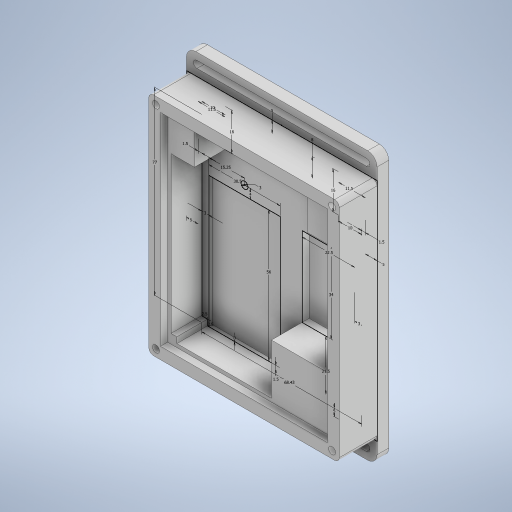
# Autodesk Inventor part: Component_shield_layered
Saved by Autodesk Inventor 2024 (Build 280153000, 153)
## iProperties
Created: 2024-10-22
Part Number: Component_shield_layered
Material: Generic
Document SubType Name: Modeling
Designer: Bruger
Density: 1 g/cm^3
Appearance: Default
Author: Bruger
Autodesk Inventor part; units mm, degrees
ref_plane "YZ Plane" through (0, 0, 0) normal (1, 0, 0) x (0, 1, 0)
ref_plane "XZ Plane" through (0, 0, 0) normal (0, 1, 0) x (-1, 0, 0)
sketch "Sketch1" plane through (0, 0, 0) normal (0, 0, 1) x (1, 0, 0)
  line L0 (0, 0) -> (68.43, 0)
  line L1 (68.43, 0) -> (68.43, 77)
  line L2 (68.43, 77) -> (0, 77)
  line L3 (0, 77) -> (0, 0)
  line L4 (3, 56) -> (33.5, 56)
  line L5 (33.5, 56) -> (33.5, 0)
  line L6 (33.5, 0) -> (3, 0)
  line L7 (3, 0) -> (3, 56)
  line L8 (42.93, 55.5) -> (65.43, 55.5)
  line L9 (65.43, 55.5) -> (65.43, 21.5)
  line L10 (65.43, 21.5) -> (42.93, 21.5)
  line L11 (42.93, 21.5) -> (42.93, 55.5)
  line L12 (-6.5, 90) -> (74.93, 90)
  line L13 (74.93, 90) -> (74.93, -6.5)
  line L14 (74.93, -6.5) -> (-6.5, -6.5)
  line L15 (-6.5, -6.5) -> (-6.5, 90)
  line L16 (-1.5, 85) -> (69.93, 85)
  line L17 (69.93, 85) -> (69.93, -1.5)
  line L18 (69.93, -1.5) -> (-1.5, -1.5)
  line L19 (-1.5, -1.5) -> (-1.5, 85)
  line L20 (42.93, 21.5) -> (68.43, 21.5)
  line L21 (68.43, 21.5) -> (68.43, 0)
  line L22 (68.43, 0) -> (42.93, 0)
  line L23 (42.93, 0) -> (42.93, 21.5)
  line L24 (0, 77) -> (10, 77)
  line L25 (68.43, 77) -> (53.43, 77)
  line L26 (68.43, 67) -> (68.43, 77)
  line L27 (0, 0) -> (2.5, 0)
  line L28 (2.5, 0) -> (2.5, 2.5)
  line L29 (2.5, 2.5) -> (0, 2.5)
  line L30 (0, 2.5) -> (0, 0)
  circle A0 centre (18.25, 60) radius 1.5
  line L31 (0, 85) -> (10, 85)
  line L32 (10, 77) -> (0, 77)
  line L33 (53.43, 77) -> (63.43, 77)
  line L34 (68.43, 85) -> (53.43, 85)
  line L35 (0, 85) -> (10, 85)
  line L36 (10, 85) -> (10, 69)
  line L37 (10, 69) -> (0, 69)
  line L38 (0, 69) -> (0, 85)
  line L39 (68.43, 85) -> (58.43, 85)
  line L40 (58.43, 85) -> (58.43, 69)
  line L41 (58.43, 69) -> (68.43, 69)
  line L42 (68.43, 69) -> (68.43, 85)
  point P0 (54.18, 21.5)
  point P1 (34.215, 90)
  point P2 (42.93, 0)
  point P3 (65.43, 21.5)
  point P4 (0, 69)
  point P5 (3, 0)
  dimension "d0" = 77
  dimension "d1" = 68.43
  dimension "d2" = 30.5
  dimension "d3" = 56
  dimension "d4" = 3
  dimension "d7" = 0
  dimension "d8" = 34
  dimension "d9" = 22.5
  dimension "d10" = 3
  dimension "d11" = 21.5
  dimension "d20" = 1.5
  dimension "d21" = 8
  dimension "d22" = 1.5
  dimension "d23" = 1.5
  dimension "d32" = 2.5
  dimension "d33" = 2.5
  dimension "d34" = 3
  dimension "d35" = 4
  dimension "d36" = 15.25
  dimension "d46" = 5
  dimension "d53" = 16
  dimension "d54" = 11.5
  dimension "d55" = 10
  dimension "d56" = 10
  dimension "d57" = 16
  dimension "d58" = 11.5
  dimension "d59" = 5
  dimension "d60" = 5
  dimension "d61" = 5
  constraints: 86 end point, 20 parallel, 13 horizontal, 9 perpendicular, 2 midpoint, 2 point on line, 1 centre point
  measures "d0" distance of L2.end L0.start
  measures "d1" distance of L0.start L0.end
  measures "d2" distance of L4.start L4.end
  measures "d3" distance of L4.end L5.end
  measures "d4" distance between parallel lines of L7 L3
  measures "d7" distance between parallel lines of L0 L6
  measures "d8" distance from line of point (54.18, 21.5) L8
  measures "d9" distance between parallel lines of L9 L11
  measures "d10" distance between parallel lines of L1 L9
  measures "d11" distance between parallel lines of L0 L10
  measures "d20" distance between parallel lines of L1 L17
  measures "d21" distance between parallel lines of L2 L16
  measures "d22" distance between parallel lines of L3 L19
  measures "d23" distance between parallel lines of L0 L18
  measures "d32" distance of L29.end L28.end
  measures "d33" distance of L28.end L27.end
  measures "d34" diameter of A0
  measures "d35" distance from line of L4 A0.centre
  measures "d36" distance from line of L7 A0.centre
  measures "d46" distance between parallel lines of L16 L12
  measures "d53" distance of L35.end L36.end
  measures "d54" distance between parallel lines of L19 L36
  measures "d55" distance between parallel lines of L36 L38
  measures "d56" distance of L41.end L40.end
  measures "d57" distance of L40.end L39.end
  measures "d58" distance between parallel lines of L17 L40
  measures "d59" distance between parallel lines of L19 L15
  measures "d60" distance between parallel lines of L18 L14
  measures "d61" distance between parallel lines of L13 L17
extrude "Extrusion1" add sketch "Sketch1" against normal blind 5 contours L3 L29 L28 L0 | L0 L1 L42 L16 L17 L18 L19 L38 L3 | L28 L29 L3 L37 L36 L2 L40 L41 L1 L20 L9 L8 L11 L23 L0 L5 L4 L7 | L7 L4 L5 L0 | L3 L2 L36 L37 | L38 L16 L36 L2 | L23 L10 L20 L1 L0 | L36 L16 L40 L2 | L11 L8 L9 L10 | L40 L16 L42 L2 | L2 L1 L41 L40 | L12 L13 L14 L15 | A0
extrude "Extrusion2" cut sketch "Sketch1" against normal blind 3 contours L11 L8 L9 L10
extrude "Extrusion5" add sketch "Sketch1" along normal blind 16.1 contours L12 L13 L14 L15
extrude "Extrusion6" add sketch "Sketch1" along normal blind 13.1 contours L3 L29 L28 L0 | L0 L1 L42 L16 L17 L18 L19 L38 L3 | L3 L2 L36 L37 | L38 L16 L36 L2 | L23 L10 L20 L1 L0 | L40 L16 L42 L2 | L2 L1 L41 L40
sketch "Sketch4" plane through (0, 0, 16.1) normal (0, 0, 1) x (1, 0, 0)
  line L0 (-1.5, -1.5) -> (-1.5, 85) projected
  line L1 (69.93, -1.5) -> (-1.5, -1.5) projected
  line L2 (74.93, -6.5) -> (-6.5, -6.5) projected
  line L3 (-1.5, -1.5) -> (-6.5, -6.5)
  line L4 (69.93, -1.5) -> (-1.5, -1.5) projected
  circle A0 centre (-1.5, -1.5) radius 2.707
  circle A1 centre (-3.4141, -3.4141) radius 1.5
  point P0 (0, 0)
  dimension "d84" = 5.414
  dimension "d85" = 3
  constraints: 2 coincident, 2 end point, 1 centre point, 1 point on line, 3 other
  measures "d85" diameter of A1
hole "Hole2" at (-3.4141, -3.4141, 16.1) direction (0, 0, -1) diameter 3 depth 10 tip angle 118
pattern_linear "Rectangular Pattern1" count 2 spacing 75.258 along (1, 0, 0) count 2 spacing 90.328 along (0, 1, 0) of "Hole2"
sketch "Sketch6" plane through (-6.5, -6.5, -5) normal (0, -1, 0) x (1, 0, 0)
  line L0 (0, 0) -> (81.43, 0) projected
  line L1 (81.43, 0) -> (81.43, 21.1) projected
  line L2 (0, 0) -> (81.43, 0)
  line L3 (81.43, 0) -> (81.43, 5)
  line L4 (81.43, 5) -> (0, 5)
  line L5 (0, 5) -> (0, 0)
  point P0 (6.5, 5)
  dimension "d86" = 5
  constraints: 8 end point, 2 parallel, 1 horizontal, 1 perpendicular, 1 point on line
  measures "d86" distance between parallel lines of L4 L0
extrude "Extrusion7" add sketch "Sketch6" along normal blind 9
sketch "Sketch7" plane through (-6.5, -6.5, 0) normal (0, 0, 1) x (1, 0, 0)
  line L0 (0, 0) -> (0, -9) construction
  line L1 (0, -4.5) -> (4.5, -4.5) construction
  circle A0 centre (4.5, -4.5) radius 1.5
  line L2 (81.43, 0) -> (81.43, -9) construction
  line L3 (81.43, -4.5) -> (76.93, -4.5) construction
  circle A1 centre (76.93, -4.5) radius 1.5
  line L4 (76.93, -6) -> (4.5, -6)
  line L5 (4.5, -3) -> (76.93, -3)
  point P0 (6.5, 6.5)
  dimension "d89" = 4.5
  dimension "d90" = 3
  dimension "d91" = 4.5
  dimension "d92" = 3
  constraints: 8 end point, 4 point on circle, 3 horizontal, 3 tangent, 2 centre point, 2 coincident, 2 midpoint
  measures "d89" distance of L1.start L1.end
  measures "d90" diameter of A0
  measures "d91" distance of L3.start L3.end
  measures "d92" diameter of A1
extrude "Extrusion8" cut sketch "Sketch7" against normal through all
fillet "Fillet3" radius 4 2 edges at (-6.5, -15.5, -2.5) (74.93, -15.5, -2.5)
ref_plane "Work Plane2" through (-6.5, 41.75, 16.1) normal (0, -1, 0) x (1, 0, 0)
mirror "Mirror2" about plane through (-6.5, 41.75, 16.1) normal (0, -1, 0) of "Extrusion8", "Extrusion7", "Fillet3"
fillet "Fillet5" radius 2 4 edges at (74.93, 90, 8.05) (-6.5, 90, 8.05) (-6.5, -6.5, 8.05) (74.93, -6.5, 8.05)
extrude "Extrusion9" cut sketch "Sketch1" against normal blind 1.5 contours L7 L4 L5 L0
body "Solid1"
